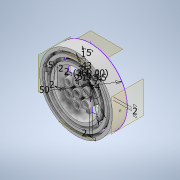
# Autodesk Inventor part: improved_gimbal
Saved by Autodesk Inventor 2021 (Build 250183000, 183)
## iProperties
Created: 2021-06-15
Part Number: improved_gimbal
Material: Generic
Document SubType Name: Modeling
Designer: Charlie
Density: 1 g/cm^3
Appearance: Default
Author: Charlie
Autodesk Inventor part; units mm, degrees
ref_plane "YZ Plane" through (0, 0, 0) normal (1, 0, 0) x (0, 1, 0)
ref_plane "XZ Plane" through (0, 0, 0) normal (0, 1, 0) x (-1, 0, 0)
ref_plane "XY Plane" through (0, 0, 0) normal (0, 0, 1) x (1, 0, 0)
sketch "Sketch1" plane through (0, 0, 0) normal (0, 0, 1) x (1, 0, 0)
  circle A0 centre (0, 0) radius 25
  circle A1 centre (0, 0) radius 23
  circle A2 centre (0, 0) radius 21.5
  circle A3 centre (0, 0) radius 19.5
  circle A4 centre (0, 0) radius 17.5
  circle A5 centre (0, 0) radius 15.5
  circle A6 centre (0, 0) radius 5
  line L0 (-0.9525, -15.4707) -> (0.9525, 15.4707) construction
  line L1 (0.9525, -15.4707) -> (-0.9525, 15.4707) construction
  circle A7 centre (0, 0) radius 2
  line L2 (-1, 15.4677) -> (-1, 4.899)
  line L3 (-1, -4.899) -> (-1, -15.4677)
  line L4 (1, -15.4677) -> (1, -4.899)
  line L5 (1, 4.899) -> (1, 15.4677)
  circle A8 centre (0, 0) radius 2.75
  circle A9 centre (0, 7) radius 2
  circle A10 centre (0, 7) radius 2.75
  line L6 (-15.4677, -1) -> (-4.899, -1)
  line L7 (4.899, -1) -> (15.4677, -1)
  line L8 (15.4677, 1) -> (4.899, 1)
  line L9 (-4.899, 1) -> (-15.4677, 1)
  circle A11 centre (-6.0622, 3.5) radius 2.75
  circle A12 centre (-6.0622, 3.5) radius 2
  circle A13 centre (-6.0622, -3.5) radius 2.75
  circle A14 centre (-6.0622, -3.5) radius 2
  circle A15 centre (0, -7) radius 2.75
  circle A16 centre (0, -7) radius 2
  circle A17 centre (6.0622, -3.5) radius 2.75
  circle A18 centre (6.0622, -3.5) radius 2
  circle A19 centre (6.0622, 3.5) radius 2.75
  circle A20 centre (6.0622, 3.5) radius 2
  circle A21 centre (0, 0) radius 9.75
  point P0 (-15, 0)
  point P1 (-25, 0)
  point P2 (25, 0)
  point P3 (0, 23)
  point P4 (0, -21.5)
  point P5 (0, 21.5)
  point P6 (-8.4437, 4.875)
  point P7 (-9.6986, 1)
  point P8 (-9.6986, -1)
  point P9 (-8.4437, -4.875)
  point P10 (-4.9165, -1)
  point P11 (-4.8971, -1.009)
  point P12 (-1, -9.6986)
  point P13 (1, -9.6986)
  point P14 (8.4437, -4.875)
  point P15 (4.8971, -1.009)
  point P16 (4.9165, -1)
  point P17 (9.6986, -1)
  point P18 (9.6986, 1)
  point P19 (8.4437, 4.875)
  point P20 (4.9165, 1)
  point P21 (4.8971, 1.009)
  point P22 (1, 9.6986)
  point P23 (-1, 9.6986)
  point P24 (-4.8971, 1.009)
  point P25 (-4.9165, 1)
  dimension "d0" = 50
  dimension "d1" = 2
  dimension "d2" = 43
  dimension "d3" = 2
  dimension "d4" = 35
  dimension "d5" = 2
  dimension "d16" = 4
  dimension "d17" = 2
  dimension "d18" = 2
  dimension "d19" = 5.5
  dimension "d48" = 4
  dimension "d49" = 5.5
  dimension "d50" = 7
  dimension "d51" = 2
  dimension "d52" = 2
  dimension "d55" = 360
  dimension "d57" = 19.5
  constraints: 20 centre point, 20 end point, 11 coincident, 8 parallel, 8 point on circle, 2 midpoint, 1 vertical alignment, 37 other
  measures "d0" diameter of A0
  measures "d2" diameter of A2
  measures "d3" radial gap between concentric circles of A2 A3
  measures "d4" diameter of A4
  measures "d16" diameter of A7
  measures "d17" distance between parallel lines of L4 L3
  measures "d18" distance between parallel lines of L2 L5
  measures "d19" diameter of A8
  measures "d48" diameter of A9
  measures "d49" diameter of A10
  measures "d50" distance of A0.centre A10.centre
  measures "d51" distance between parallel lines of L8 L7
  measures "d52" distance between parallel lines of L6 L9
  measures "d57" diameter of A21
extrude "Extrusion1" add sketch "Sketch1" along normal blind 10 contours A0
ref_plane "Work Plane1" through (-25, 0, 0) normal (-1, 0, 0) x (0, -1, 0)
sketch "Sketch2" plane through (-25, 0, 0) normal (-1, 0, 0) x (0, -1, 0)
  line L0 (0, 0) -> (0, 5)
  circle A0 centre (0, 5) radius 0.5
  dimension "d22" = 5
  dimension "d23" = 1
  constraints: 2 end point, 1 centre point, 1 coincident, 1 vertical
  measures "d22" distance of L0.start L0.end
  measures "d23" diameter of A0
extrude "Extrusion2" cut sketch "Sketch2" against normal blind 50
extrude "Extrusion3" add sketch "Sketch1" along normal blind 10 contours A2
ref_plane "Work Plane2" through (0, 21.5, 0) normal (0, 1, 0) x (-1, 0, 0)
sketch "Sketch3" plane through (0, 21.5, 0) normal (0, 1, 0) x (-1, 0, 0)
  line L0 (0, 0) -> (0, 5)
  circle A0 centre (0, 5) radius 0.5
  dimension "d28" = 5
  dimension "d29" = 1
  constraints: 2 end point, 1 centre point, 1 coincident, 1 vertical
  measures "d28" distance of L0.start L0.end
  measures "d29" diameter of A0
extrude "Extrusion4" cut sketch "Sketch3" against normal blind 44
extrude "Extrusion5" cut sketch "Sketch2" against normal blind 4.5
ref_plane "Work Plane3" through (25, 0, 0) normal (1, 0, 0) x (0, 1, 0)
sketch "Sketch4" plane through (25, 0, 0) normal (1, 0, 0) x (0, 1, 0)
  circle A0 centre (0, 5) radius 0.5 projected
  circle A1 centre (0, 5) radius 0.5
  point P0 (0, 0)
  dimension "d34" = 1
  constraints: 1 centre point, 1 coincident
  measures "d34" diameter of A1
extrude "Extrusion6" cut sketch "Sketch4" against normal blind 4.5
extrude "Extrusion7" add sketch "Sketch1" along normal blind 10 contours A4
extrude "Extrusion8" cut sketch "Sketch3" against normal blind 5
ref_plane "Work Plane4" through (0, -21.5, 0) normal (0, -1, 0) x (1, 0, 0)
sketch "Sketch5" plane through (0, -21.5, 0) normal (0, -1, 0) x (1, 0, 0)
  circle A0 centre (0, 5) radius 0.5 projected
  circle A1 centre (0, 5) radius 0.5
  point P0 (0, 0)
  dimension "d41" = 1
  constraints: 1 centre point, 1 coincident
  measures "d41" diameter of A1
extrude "Extrusion9" cut sketch "Sketch5" against normal blind 5
extrude "Extrusion10" add sketch "Sketch1" along normal blind 2 contours A5 L7 A21 L8 | L5 A21 L2 A5 | A21 L7 A17 A6 L8 A19 | L8 A19 A21 | A5 L3 A21 L4 | A21 A17 L7 | A21 A19 A6 A10 L5 | L5 A10 A21 | A21 A15 L4 | L4 A15 A6 A17 A21 | L9 A21 L6 A5 | A21 A10 L2 | L2 A10 A6 A11 A21 | A19 A6 A17 A15 A13 A11 A10 | A21 A13 A6 A15 L3 | L3 A15 A21 | A21 A11 L9 | L9 A11 A6 L6 A13 A21 | L6 A13 A21
extrude "Extrusion11" add sketch "Sketch1" along normal blind 10 contours A19 L8 | L8 A19 A6 | A17 A6 L7 | L7 A17 | A10 A6 L5 A9 | L5 A9 L2 A10 | A6 A19 | A15 L3 A16 L4 | L4 A16 A6 A15 | A17 A6 | L2 A9 A6 A10 | A11 A6 L9 | A10 A6 | A15 A6 L3 A16 | A13 L6 A6 | A6 A15 | L9 A11 | A11 A6 | L5 A6 A9 | A13 L6 | A6 A13 | A16 A6 L4 | A9 A6 L2 | L3 A6 A16 | A8 picked at (5.9988, 1.1697) picked at (5.9988, -1.1697) picked at (-6.0041, 1.1692) picked at (-6.0041, -1.1692)
body "Solid1"
